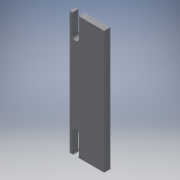
# Autodesk Inventor part: Belt_bridge
Saved by Autodesk Inventor 2019.3 (Build 233278000, 278)
## iProperties
Created: 2020-09-08
Part Number: Belt_bridge
Material: Generisch
Document SubType Name: Modeling
Designer: Nicolas Frick
Density: 1 g/cm^3
Appearance: Vorgabe
Author: Nicolas Frick
Autodesk Inventor part; units mm, degrees
ref_plane "YZ Plane" through (0, 0, 0) normal (1, 0, 0) x (0, 1, 0)
ref_plane "XZ Plane" through (0, 0, 0) normal (0, 1, 0) x (-1, 0, 0)
ref_plane "XY Plane" through (0, 0, 0) normal (0, 0, 1) x (1, 0, 0)
sketch "Skizze1" plane through (0, 0, 0) normal (0, 0, 1) x (1, 0, 0)
  line L0 (-16.9054, -20.4011) -> (0, -20.4011) construction
  line L1 (-16.9054, -20.4011) -> (-16.9054, -35)
  line L2 (-16.9054, -35) -> (0, -35) construction
  line L3 (0, -35) -> (0, -20.4011)
  line L4 (-16.9054, 10.4011) -> (0, 10.4011) construction
  line L5 (0, 25) -> (0, 10.4011)
  line L6 (-16.9054, 25) -> (0, 25)
  line L7 (-16.9054, 10.4011) -> (-16.9054, 25)
  circle A0 centre (-13.9737, 15.4205) radius 1.6 construction
  circle A1 centre (-13.9737, 21.411) radius 1.6 construction
  line L8 (0, -35) -> (0, 25)
  line L9 (-16.9054, 25) -> (-16.9054, -35)
  circle A2 centre (-13.9737, -33.881) radius 1.6 construction
  circle A3 centre (-13.9737, -27.8905) radius 1.6 construction
  line L10 (-3.735, -37.47) -> (-3.735, -22.8711) construction
  line L11 (-14.7766, -37.47) -> (-3.735, -37.47) construction
  spline S0 degree 3 poles (-16.9054, -39.47) (-16.9054, -39.2281) (-16.8461, -38.944) (-16.6519, -38.4921) (-16.4798, -38.2465) (-16.1125, -37.8931) (-15.8497, -37.7256) (-15.3599, -37.53) (-15.0443, -37.47) (-14.7766, -37.47) knots 0 0 0 0 0.237315 0.237315 0.482541 0.482541 0.737375 0.737375 1 1 1 1 construction
  line L12 (-16.9054, -22.8711) -> (-16.9054, -39.47) construction
  line L13 (-16.9054, -22.8711) -> (-3.735, -22.8711) construction
  line L14 (-16.9054, 25) -> (-16.9054, -35)
  line L15 (0, -35) -> (0, 25)
  line L16 (-13.9737, 15.4205) -> (-13.9737, 25) construction
  line L17 (-12.3737, 15.4205) -> (-12.3737, 25)
  line L18 (-15.5737, 25) -> (-15.5737, 15.4205)
  arc A4 (-15.5737, 15.4205) -> (-12.3737, 15.4205) centre (-13.9737, 15.4205) ccw
  line L19 (-13.9737, -33.881) -> (-13.9737, -24.6914) construction
  line L20 (-12.3737, -33.881) -> (-12.3737, -24.6914)
  line L21 (-15.5737, -24.6914) -> (-15.5737, -33.881)
  arc A5 (-12.3737, -24.6914) -> (-15.5737, -24.6914) centre (-13.9737, -24.6914) ccw
  arc A6 (-15.5737, -33.881) -> (-15.1173, -35) centre (-13.9737, -33.881) ccw
  arc A7 (-12.8301, -35) -> (-12.3737, -33.881) centre (-13.9737, -33.881) ccw
  line L22 (0, 25) -> (-12.3737, 25)
  line L23 (-15.5737, 25) -> (-16.9054, 25)
  line L24 (0, 25) -> (-12.3737, 25)
  line L25 (-15.5737, 25) -> (-16.9054, 25)
  line L26 (0, -35) -> (-12.8301, -35)
  line L27 (-15.1173, -35) -> (-16.9054, -35)
  point P0 (0, 0)
  point P1 (-16.9054, -37.3)
  point P2 (-13.9737, 20.2103)
  point P3 (-13.9737, -29.2862)
  dimension "d7" = 3.2
  constraints: 36 end point, 8 point on circle, 6 tangent, 4 centre point, 4 parallel, 3 perpendicular, 2 collinear, 2 horizontal, 2 midpoint, 1 point on line, 1 vertical
  measures "d7" diameter of A5
extrude "Extrusion3" add sketch "Skizze1" along normal blind 3 contours L9 L7 L6 L18 A4 L17 L5 L8 L3 L26 A7 L20 A5 L21 A6 L27 L1
